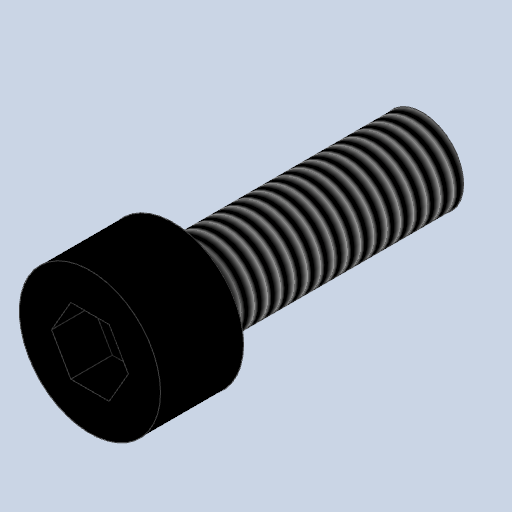
# Autodesk Inventor part: FC-0515EB
Saved by Autodesk Inventor 2022 (Build 260153000, 153)
## iProperties
Part Number: FC-0515EB
Material: ステンレス鋼 AISI 304
Document SubType Name: Modeling
Designer: Masato Kubotera
Density: 1.14237 g/cm^3
Appearance: 陽極酸化 - 黒
Mass: 0.621 g
Surface Area: 5.17268 cm^2
Volume: 0.543608 cm^3
Description: ReadyMade
Catalog Web Link: https://wilco.jp/products/F/FC-EB.html
Author: Masato Kubotera
Comments: Width across flats : 4
Autodesk Inventor part; units mm, degrees
ref_plane "YZ Plane" through (0, 0, 0) normal (1, 0, 0) x (0, 1, 0)
ref_plane "XZ Plane" through (0, 0, 0) normal (0, 1, 0) x (-1, 0, 0)
ref_plane "XY Plane" through (0, 0, 0) normal (0, 0, 1) x (1, 0, 0)
sketch "スケッチ1" plane through (0, 0, 0) normal (1, 0, 0) x (0, 1, 0)
  line L0 (0, 20) -> (0, 0)
  line L1 (0, 0) -> (4.25, 0)
  line L2 (4.25, 0) -> (4.25, 5)
  line L3 (4.25, 5) -> (2.5, 5)
  line L4 (2.5, 5) -> (2.5, 20)
  line L5 (2.5, 20) -> (0, 20)
  dimension "d2" = 5
  dimension "d10" = 15
  dimension "d11" = 5
  dimension "d12" = 8.5
  constraints: 12 end point, 5 perpendicular, 1 vertical
  measures "d2" distance of L1.end L2.end
  measures "d10" distance of L3.end L4.end
  measures "d11" diameter of L4 L0
  measures "d12" diameter of L2 L0
revolve "回転1" add sketch "スケッチ1" angle 360 about axis through (0, 0, 20) along (0, 0, -1)
thread "ねじ1" size "M5x0.8" class "6g" standard "ANSI Metric M Profile" full length
sketch "スケッチ2" plane through (0, 0, 0) normal (0, 0, -1) x (-1, 0, 0)
  line L0 (0, 2.3094) -> (2, 1.1547)
  line L1 (2, 1.1547) -> (2, -1.1547)
  line L2 (2, -1.1547) -> (0, -2.3094)
  line L3 (0, -2.3094) -> (-2, -1.1547)
  line L4 (-2, -1.1547) -> (-2, 1.1547)
  line L5 (-2, 1.1547) -> (0, 2.3094)
  circle A0 centre (0, 0) radius 4.25 projected
  line L6 (0, 4.25) -> (0, -4.25) construction
  dimension "d7" = 4
  constraints: 14 end point, 2 point on circle, 1 coincident, 1 midpoint, 1 point on line, 1 vertical, 13 other
  measures "d7" distance between parallel lines of L1 L4
extrude "押し出し1" cut sketch "スケッチ2" against normal blind 2.5 contours L0 L1 L2 L3 L4 L5
